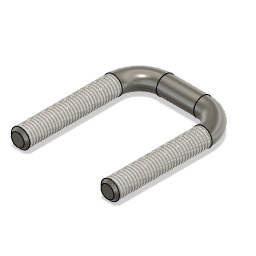
0.885.6041 - Etrier de fixation hauban - IGTE 21400_17 Rep. 53 (Autodesk Fusion 360 design; units mm, degrees)
Autodesk Fusion 360 part; units mm, degrees
sketch "Sketch1" plane through (0, 0, 0) normal (0, 0, 1) x (1, 0, 0)
  line L0 (0, 0) -> (24, 0) construction
  line L1 (0, 0) -> (-24, 0) construction
  circle A0 centre (-24, 0) radius 5
  circle A1 centre (24, 0) radius 5
  dimension "d1" = 24
  dimension "d2" = 24
  dimension "d3" = 10
  dimension "d4" = 10
  constraint coincident L0.start L1.start
  constraint coincident L1.end A0.centre
  constraint coincident L0.end A1.centre
  measures "d1" distance of L0.start L0.end
  measures "d2" distance of L0.start L1.end
  measures "d3" diameter of A0
  measures "d4" diameter of A1
extrude "Extrude1" add sketch "Sketch1" along normal blind 50 makes body 1 at (-19.0248, -0.4978, 16.6667) makes body 2 at (28.9752, -0.4978, 16.6667)
sketch "Sketch2" plane through (0, 0, 0) normal (0, 1, 0) x (1, 0, 0)
  line L0 (0, 0) -> (0, 15) construction
  line L1 (0, 15) -> (10, 15)
  line L2 (19, 0) -> (29, 0)
  line L3 (24, 0) -> (24, 1)
  line L4 (-29, 0) -> (-19, 0)
  line L5 (-24, 0) -> (-24, 1)
  line L6 (0, 15) -> (-10, 15)
  arc A0 (-10, 15) -> (-24, 1) centre (-10, 1) ccw
  arc A1 (24, 1) -> (10, 15) centre (10, 1) ccw
  dimension "d7" = 15
  dimension "d9" = 14
  dimension "d10" = 14
  constraint coincident L0.start origin
  constraint perpendicular L0 L1
  constraint midpoint L2 L3.start
  constraint perpendicular L1 L3
  constraint midpoint L4 L5.start
  constraint perpendicular L4 L5
  constraint perpendicular L0 L6
  constraint tangent L5 A0
  constraint tangent L6 A0
  constraint tangent L1 A1
  constraint tangent L3 A1
  measures "d7" distance of L0.start L0.end
  measures "d9" radius of A0
  measures "d10" radius of A1
sweep "Sweep1" add 1 faces at (-22.7139, -0.2755, 0) path "Sketch2" along L3 A1 L1 L6 A0 L5 on bodies 1 bodies 1 2
thread "Thread1" "ISO Metric profile 10.0 M10x1.5 6g" major diameter 9.85 minor diameter 8.141 pitch 1.5 angle 60 resizes the face on face at (-19.0248, 0.4978, 16) on bodies 1
thread "Thread2" "ISO Metric profile 10.0 M10x1.5 6g" major diameter 9.85 minor diameter 8.141 pitch 1.5 angle 60 resizes the face on face at (28.9005, -0.4904, -0.3333) on face at (28.9005, -0.4904, 16.6667) on bodies 1
chamfer "Chamfer1" distance 1.5 angle 45 2 edges at (-28.5917, -1.781, 50) (28.5917, 1.781, 50) on bodies 1
